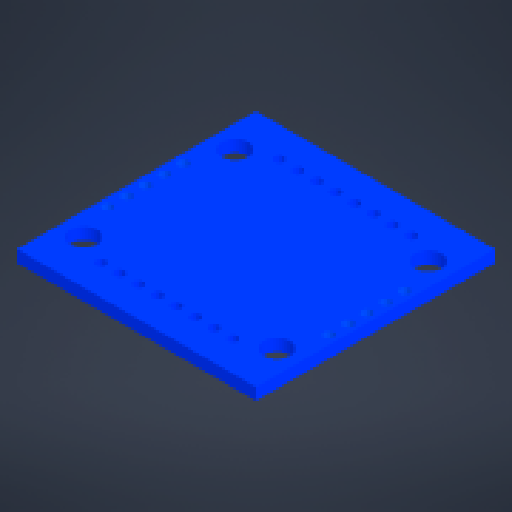
# Autodesk Inventor part: PCB
Saved by Autodesk Inventor 2025.2 (Build 292293000, 293)
## iProperties
Created: 2025-06-28
Part Number: PCB
Material: Generic
Document SubType Name: Modeling
Designer: micyg
Density: 1 g/cm^3
Appearance: Default
Author: micyg
Autodesk Inventor part; units mm, degrees
ref_plane "YZ Plane" through (0, 0, 0) normal (1, 0, 0) x (0, 1, 0)
ref_plane "XZ Plane" through (0, 0, 0) normal (0, 1, 0) x (-1, 0, 0)
ref_plane "XY Plane" through (0, 0, 0) normal (0, 0, 1) x (1, 0, 0)
sketch "Sketch1" plane through (0, 0, 0) normal (0, 1, 0) x (-1, 0, 0)
  line L0 (0, 0) -> (32.15, 0)
  line L1 (32.15, 0) -> (32.15, -32.15)
  line L2 (32.15, -32.15) -> (0, -32.15)
  line L3 (0, -32.15) -> (0, 0)
  circle A0 centre (29.0575, -5.89) radius 1.75
  circle A1 centre (29.0575, -26.26) radius 1.75
  line L4 (32.15, -16.075) -> (0, -16.075) construction
  line L5 (29.0575, -5.89) -> (3.0925, -5.89) construction
  line L6 (3.0925, -5.89) -> (3.0925, -26.26) construction
  line L7 (3.0925, -26.26) -> (29.0575, -26.26) construction
  line L8 (29.0575, -26.26) -> (29.0575, -5.89) construction
  circle A2 centre (3.0925, -5.89) radius 1.75
  circle A3 centre (3.0925, -26.26) radius 1.75
  line L9 (29.0575, -5.89) -> (3.0925, -26.26) construction
  circle A4 centre (24.965, -28.075) radius 0.635
  circle A5 centre (22.425, -28.075) radius 0.635
  circle A6 centre (19.885, -28.075) radius 0.635
  circle A7 centre (17.345, -28.075) radius 0.635
  circle A8 centre (14.805, -28.075) radius 0.635
  circle A9 centre (12.265, -28.075) radius 0.635
  circle A10 centre (9.725, -28.075) radius 0.635
  circle A11 centre (7.185, -28.075) radius 0.635
  circle A12 centre (24.965, -4.075) radius 0.635
  circle A13 centre (22.425, -4.075) radius 0.635
  circle A14 centre (19.885, -4.075) radius 0.635
  circle A15 centre (17.345, -4.075) radius 0.635
  circle A16 centre (14.805, -4.075) radius 0.635
  circle A17 centre (12.265, -4.075) radius 0.635
  circle A18 centre (9.725, -4.075) radius 0.635
  circle A19 centre (7.185, -4.075) radius 0.635
  line L10 (24.965, -4.075) -> (7.185, -28.075) construction
  circle A20 centre (30.9625, -21.155) radius 0.635
  circle A21 centre (30.9625, -18.615) radius 0.635
  circle A22 centre (30.9625, -16.075) radius 0.635
  circle A23 centre (30.9625, -13.535) radius 0.635
  circle A24 centre (30.9625, -10.995) radius 0.635
  circle A25 centre (1.1875, -21.155) radius 0.635
  circle A26 centre (1.1875, -18.615) radius 0.635
  circle A27 centre (1.1875, -16.075) radius 0.635
  circle A28 centre (1.1875, -13.535) radius 0.635
  circle A29 centre (1.1875, -10.995) radius 0.635
  line L11 (30.9625, -21.155) -> (1.1875, -10.995) construction
  point P0 (29.0575, -16.075)
  point P1 (16.075, -16.075)
  dimension "d0" = 32.15
  dimension "d1" = 32.15
  dimension "d3" = 20.37
  dimension "d4" = 3.5
  dimension "d5" = 3.5
  dimension "d6" = 3.5
  dimension "d7" = 3.5
  dimension "d8" = 25.965
  dimension "d9" = 1.27
  dimension "d12" = 2.54
  dimension "d15" = 24
  dimension "d20" = 1.27
  dimension "d23" = 2.54
  dimension "d26" = 29.775
  constraints: 30 centre point, 24 end point, 7 midpoint, 4 coincident, 4 horizontal, 4 parallel, 2 perpendicular, 2 vertical, 1 point on line, 48 other
  measures "d0" distance of L1.end L2.end
  measures "d1" distance of L0.end L1.end
  measures "d3" distance of L7.end L5.start
  measures "d4" diameter of A0
  measures "d5" diameter of A1
  measures "d6" diameter of A3
  measures "d7" diameter of A2
  measures "d8" distance of L6.end L7.end
  measures "d9" diameter of A4
  measures "d12" distance of A4.centre A5.centre
  measures "d15" distance of A4.centre L10.start
  measures "d20" diameter of A20
  measures "d23" distance of L11.start A21.centre
  measures "d26" distance of L11.start A25.centre
extrude "Extrusion1" add sketch "Sketch1" along normal blind 1.6
equation "\"d5\" = d4"
equation "\"d6\" = d4"
equation "\"d7\" = d4"
equation "\"d20\" = d9"
body "Solid1"
